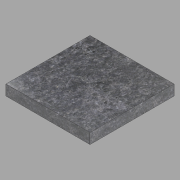
# Autodesk Inventor part: 16x16x2 - 14
Saved by Autodesk Inventor 2022.2 (Build 262287000, 287)
## iProperties
Created: 2022-03-01
Part Number: 16x16x2 - 14
Material: Granite, Cut, Polished
Document SubType Name: Modeling
Designer: awelt
Mass: 22653.5 g
Surface Area: 4129.02 cm^2
Volume: 8390.18 cm^3
Density: 2.7 g/cm^3
Appearance: Kasota SN sapphire
Author: awelt
Autodesk Inventor part; units mm, degrees
ref_plane "YZ Plane" through (0, 0, 0) normal (1, 0, 0) x (0, 1, 0)
ref_plane "XZ Plane" through (0, 0, 0) normal (0, 1, 0) x (-1, 0, 0)
ref_plane "XY Plane" through (0, 0, 0) normal (0, 0, 1) x (1, 0, 0)
sketch "Sketch1" plane through (0, 0, 0) normal (0, 1, 0) x (-1, 0, 0)
  line L0 (203.2, -203.2) -> (-203.2, -203.2)
  line L1 (-203.2, -203.2) -> (-203.2, 203.2)
  line L2 (-203.2, 203.2) -> (203.2, 203.2)
  line L3 (203.2, 203.2) -> (203.2, -203.2)
  line L4 (203.2, -203.2) -> (-203.2, 203.2) construction
  line L5 (-203.2, -203.2) -> (203.2, 203.2) construction
  point P0 (0, 0)
  dimension "d0" = 406.4
  dimension "d1" = 406.4
  constraints: 12 end point, 2 midpoint, 2 parallel, 1 horizontal, 1 perpendicular
  measures "d0" distance of L1.end L2.end
  measures "d1" distance of L0.end L1.end
extrude "Extrusion1" add sketch "Sketch1" along normal blind 50.8
body "Solid1"
